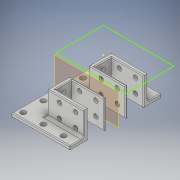
# Autodesk Inventor part: Base holder
Saved by Autodesk Inventor 2018 (Build 220112000, 112)
## iProperties
Created: 2018-09-29
Part Number: Base holder
Material: Generic
Document SubType Name: Modeling
Designer: Iek Man Lei
Density: 1 g/cm^3
Appearance: Default
Author: Iek Man Lei
Autodesk Inventor part; units mm, degrees
ref_plane "YZ Plane" through (0, 0, 0) normal (1, 0, 0) x (0, 1, 0)
ref_plane "XZ Plane" through (0, 0, 0) normal (0, 1, 0) x (-1, 0, 0)
sketch "Sketch1" plane through (0, 0, 0) normal (0, 1, 0) x (-1, 0, 0)
  line L0 (24.7222, 19.7778) -> (-57.2778, 19.7778)
  line L1 (-57.2778, 19.7778) -> (-57.2778, -24.7222)
  line L2 (-57.2778, -24.7222) -> (24.7222, -24.7222)
  line L3 (24.7222, -24.7222) -> (24.7222, 19.7778)
  circle A0 centre (17.7222, 7.2778) radius 3.3
  circle A1 centre (17.7222, -17.7222) radius 3.3
  circle A2 centre (-7.2778, 7.2778) radius 3.3
  circle A3 centre (-7.2778, -17.7222) radius 3.3
  circle A4 centre (17.7222, -17.7222) radius 3.3
  circle A5 centre (-7.2778, 7.2778) radius 3.3
  circle A6 centre (-7.2778, -17.7222) radius 3.3
  circle A7 centre (-32.2778, 7.2778) radius 3.3
  circle A8 centre (-32.2778, -17.7222) radius 3.3
  line L4 (-7.2778, 17.2778) -> (-57.2778, 17.2778)
  line L5 (-57.2778, 17.2778) -> (-57.2778, -2.7222)
  line L6 (-57.2778, -2.7222) -> (-7.2778, -2.7222)
  line L7 (-7.2778, -2.7222) -> (-7.2778, 17.2778)
  point P0 (0, 0)
  dimension "d0" = 44.5
  dimension "d1" = 82
  dimension "d2" = 6.6
  dimension "d3" = 12.5
  dimension "d4" = 7
  dimension "d7" = 25
  dimension "d10" = 25
  dimension "d15" = 25
  dimension "d18" = 25
  dimension "d21" = 50
  dimension "d22" = 20
  dimension "d23" = 0
  dimension "d24" = 10
  constraints: 16 end point, 9 centre point, 4 horizontal, 4 parallel, 2 perpendicular, 2 vertical, 16 other
  measures "d0" distance of L2.end L0.start
  measures "d1" distance of L1.end L2.end
  measures "d2" diameter of A0
  measures "d3" distance from line of L0 A0.centre
  measures "d4" distance from line of L3 A0.centre
  measures "d7" distance of A0.centre A1.centre
  measures "d10" distance of A0.centre A2.centre
  measures "d15" distance of A0.centre A4.centre
  measures "d18" distance of A0.centre A5.centre
  measures "d21" distance of L6.end L5.end
  measures "d22" distance of L4.end L5.end
  measures "d23" distance between parallel lines of L1 L5
  measures "d24" distance from line of L4 A7.centre
extrude "Extrusion1" add sketch "Sketch1" along normal blind 5 contours L3 L2 L1 L6 L7 A2 L4 L0 | L7 A2 | A2 L7
sketch "Sketch2" plane through (0, 5, 0) normal (0, 1, 0) x (1, 0, 0)
  line L0 (57.2778, 2.7222) -> (57.2778, 24.7222) projected
  line L1 (-24.7222, -19.7778) -> (57.2778, -19.7778) projected
  line L2 (57.2778, 24.7222) -> (47.2778, 24.7222)
  line L3 (47.2778, 24.7222) -> (47.2778, -19.7778)
  line L4 (47.2778, -19.7778) -> (57.2778, -19.7778)
  line L5 (57.2778, -19.7778) -> (57.2778, 24.7222)
  point P0 (0, 0)
  dimension "d27" = 10
  constraints: 8 end point, 2 parallel, 1 horizontal, 1 perpendicular, 1 point on line
  measures "d27" distance of L4.end L3.end
extrude "Extrusion2" cut sketch "Sketch2" against normal blind 5
sketch "Sketch3" plane through (0, 5, 0) normal (0, 1, 0) x (1, 0, 0)
  line L0 (7.2778, -10.5778) -> (7.2778, -17.2778) projected
  line L1 (7.2778, -12.7) -> (12.7, -12.7)
  line L2 (12.7, -12.7) -> (12.7, 0)
  line L3 (12.7, 0) -> (7.2778, 0)
  line L4 (7.2778, 0) -> (7.2778, -12.7)
  point P0 (0, 0)
  constraints: 8 end point, 2 parallel, 1 horizontal, 1 perpendicular, 1 point on line
extrude "Extrusion3" cut sketch "Sketch3" against normal blind 5
sketch "Sketch4" plane through (0, 5, 0) normal (0, 1, 0) x (1, 0, 0)
  line L0 (47.2778, 24.7222) -> (47.2778, 2.7222) projected
  line L1 (47.2778, 2.7222) -> (7.2778, 2.7222)
  line L2 (7.2778, 2.7222) -> (7.2778, 7.7222)
  line L3 (7.2778, 7.7222) -> (47.2778, 7.7222)
  line L4 (47.2778, 7.7222) -> (47.2778, 2.7222)
  point P0 (0, 0)
  dimension "d32" = 40
  dimension "d33" = 5
  constraints: 8 end point, 2 parallel, 1 horizontal, 1 perpendicular
  measures "d32" distance of L2.end L3.end
  measures "d33" distance of L1.end L2.end
extrude "Extrusion4" add sketch "Sketch4" along normal blind 30
sketch "Sketch5" plane through (0, 5, 0) normal (0, 1, 0) x (1, 0, 0)
  line L0 (7.2778, 2.7222) -> (7.2778, 7.7222) projected
  line L1 (7.2778, 7.7222) -> (2.2778, 7.7222)
  line L2 (2.2778, 7.7222) -> (2.2778, -17.2778)
  line L3 (2.2778, -17.2778) -> (7.2778, -17.2778)
  line L4 (7.2778, -17.2778) -> (7.2778, 7.7222)
  point P0 (0, 0)
  dimension "d36" = 5
  dimension "d37" = 25
  constraints: 8 end point, 2 parallel, 1 horizontal, 1 perpendicular
  measures "d36" distance of L3.end L2.end
  measures "d37" distance of L3.end L0.end
extrude "Extrusion5" add sketch "Sketch5" along normal blind 30
sketch "Sketch6" plane through (0, 5, 0) normal (0, 1, 0) x (1, 0, 0)
  line L0 (-24.7222, -19.7778) -> (47.2778, -19.7778) projected
  line L1 (47.2778, -17.2778) -> (2.2778, -17.2778)
  line L2 (2.2778, -17.2778) -> (2.2778, -19.7778)
  line L3 (2.2778, -19.7778) -> (47.2778, -19.7778)
  line L4 (47.2778, -19.7778) -> (47.2778, -17.2778)
  point P0 (0, 0)
  dimension "d40" = 45
  dimension "d43" = 2.5
  constraints: 8 end point, 2 parallel, 1 horizontal, 1 perpendicular, 1 point on line
  measures "d40" distance of L3.end L2.end
  measures "d43" distance of L1.end L2.end
extrude "Extrusion6" add sketch "Sketch6" along normal blind 30
sketch "Sketch7" plane through (2.2778, 5, -7.7222) normal (-1, 0, 0) x (0, 0, 1)
  circle A0 centre (15, 6.35) radius 2.75
  circle A1 centre (15, 21.3418) radius 2.75
  line L0 (5, -5) -> (5, 30) projected
  point P0 (7.7222, -5)
  dimension "d44" = 5.5
  dimension "d45" = 5.5
  dimension "d46" = 10
  constraints: 2 centre point, 1 vertical alignment
  measures "d44" diameter of A0
  measures "d45" diameter of A1
  measures "d46" distance from line of L0 A1.centre
extrude "Extrusion7" cut sketch "Sketch7" against normal blind 30
sketch "Sketch8" plane through (-24.7222, 0, 19.7778) normal (0, 0, 1) x (1, 0, 0)
  circle A0 centre (42, 11) radius 2.75
  circle A1 centre (62, 11) radius 2.75
  circle A2 centre (42, 28) radius 2.75
  circle A3 centre (62, 28) radius 2.75
  line L0 (32, 0) -> (32, 35) projected
  line L1 (72, 0) -> (72, 35) projected
  line L2 (27, 35) -> (72, 35) projected
  point P0 (24.7222, 0)
  dimension "d49" = 5.5
  dimension "d50" = 5.5
  dimension "d51" = 5.5
  dimension "d52" = 5.5
  dimension "d53" = 10
  dimension "d54" = 10
  dimension "d55" = 17
  dimension "d56" = 7
  constraints: 4 centre point, 2 horizontal alignment, 2 vertical alignment
  measures "d49" diameter of A0
  measures "d50" diameter of A1
  measures "d51" diameter of A2
  measures "d52" diameter of A3
  measures "d53" distance from line of L0 A2.centre
  measures "d54" distance from line of L1 A3.centre
  measures "d55" distance of A1.centre A3.centre
  measures "d56" distance from line of L2 A3.centre
extrude "Extrusion8" cut sketch "Sketch8" against normal through all
fillet "Fillet1" radius 3 2 edges at (24.7778, 5, -7.7222) (2.2778, 5, 6.0278)
fillet "Fillet2" radius 1 27 edges at (47.2778, 5.8787, -8.6009) (47.2778, 5, -17.7222) (47.2778, 21.5, -7.7222) (47.2778, 17.5, -2.7222) (27.2778, 35, -2.7222) (24.7778, 35, -7.7222) (7.2778, 35, 7.2778) (2.2778, 35, 6.0278) (27.2778, 35, 17.2778) (24.7778, 35, 19.7778) (47.2778, 17.5, 19.7778) (47.2778, 17.5, 17.2778) (47.2778, 0, -13.7222) (27.2778, 0, -2.7222) (11.2778, 0, 19.7778) (2.2778, 21.5, 19.7778) (-12.7222, 5, 19.7778) (1.3991, 5.8787, 19.7778) (-24.7222, 5, -2.4722) (11.2778, 5, -24.7222) (11.2778, 0, -24.7222) (47.2778, 2.5, -24.7222) (-24.7222, 0, -2.4722) (7.2778, 0, 7.2778) (27.2778, 0, 17.2778) (1.3991, 5.8787, -8.6009) (2.2778, 21.5, -7.7222)
ref_plane "Work Plane1" through (0, 0, 31.75) normal (0, 0, 1) x (1, 0, 0)
mirror "Mirror1" about plane through (0, 0, 31.75) normal (0, 0, 1) of "Fillet2", "Extrusion1", "Extrusion6", "Fillet1", "Extrusion4", "Extrusion5", "Extrusion3", "Extrusion2", "Extrusion8", "Extrusion7"
sketch "Sketch9" plane through (0, 35, 0) normal (0, 1, 0) x (1, 0, 0)
  line L0 (55.5625, 31.75) -> (-31.75, 31.75)
  line L1 (-31.75, 31.75) -> (-31.75, -26.9875)
  line L2 (-31.75, -26.9875) -> (55.5625, -26.9875)
  line L3 (55.5625, -26.9875) -> (55.5625, 31.75)
  point P0 (0, 0)
  constraints: 8 end point, 2 parallel, 1 horizontal, 1 perpendicular
body "Solid1"
